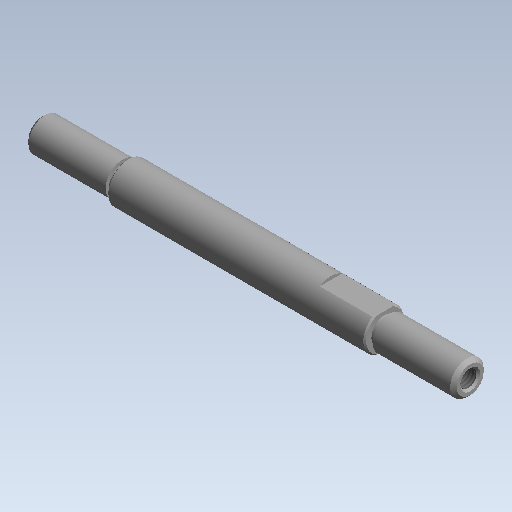
# Autodesk Inventor part: SSFRMHHS6-38.3-F12.7-P5-T12.7-M3-SC0-TF12.7-TT12.7
Saved by Autodesk Inventor 2020.3 (Build 243373000, 373)
## iProperties
Part Number: SSFRMHHS6-38.3-F12.7-P5-T12.7-M3-SC0-TF12.7-TT12.7
Material: 一般
Catalog Web Link: www.cadenas.de
Description: NSFRMHHS, SFRMHHS, PSFRMHHS, SSFRMHHS, NSFRMGHS, SFRMGHS, PSFRMGHS, SSFRMGHS, NSFRHHS, SFRHHS, PSFRHHS, SSFRHHS, NSFRHS, SFRHS, PSFRHS, SSFRHS_shaft-Rotary Shafts - Both Ends Stepped and Tapped - Wrench Flats
Vendor: MISUMI
Document SubType Name: Modeling
Designer: partserver
Manufacturer: MISUMI
Mass: 1.45427 g
Surface Area: 13.2412 cm^2
Volume: 1.45427 cm^3
Density: 1 g/cm^3
Appearance: PSOLRGB-192-192-192
Category: PARTsolutions
Company: MISUMI
PSOL_IDENT_0: {$CADENAS_DATA\23d-libs\misumi\metric\11_rotary_shafts\11_components\psfrhs\psfrhs.prj},734 {VTYP=3D
PSOL_IDENT_1: },{NB=SSFRMHHS6-38.3-F12.7-P5-T12.7-M3-SC0_s},{LINA=SSFRMHHS6-38.3-F12.7-P5-T12.7-M3-SC0},{NN=NSFRMH
PSOL_IDENT_2: HS, SFRMHHS, PSFRMHHS, SSFRMHHS, NSFRMGHS, SFRMGHS, PSFRMGHS, SSFRMGHS, NSFRHHS, SFRHHS, PSFRHHS, SS
PSOL_IDENT_3: FRHHS, NSFRHS, SFRHS, PSFRHS, SSFRHS_shaft},{DATE=11.03.2021 14:31:30},{GEOMDATE=16.02.2021 10:15:52
PSOL_IDENT_4: },{VERSION=},{LINEID=110},{WBVAR=TS,TYS,MAT,ST,ALT1,L,ALT9,F,T,P,M,SC,ALT2,KC,A,WKC,C,K,E,KZ,Z,ALT8,
PSOL_IDENT_5: PKC,ALT14,QKC,ALT21,PP,PK,ALT23,PV,PW,ALT22,QQ,QK,ALT24,QV,QW,ALT27,TL,TR,ALT28,TF,ALT29,TTALT29,ALT
PSOL_IDENT_6: 3,FC,GALT3,WFC,J,WALT3,V,ALT4,SFC,SG,AG,ALT25,PFC,LC,ALT26,QFC,RC,ALT5,UC,ALT31},{WBNUMERIC=L,F,T,P,
PSOL_IDENT_7: M,SC,KC,A,WKC,C,K,E,KZ,Z,PKC,QKC,PP,PK,PV,PW,QQ,QK,QV,QW,TL,TR,TF,TTALT29,FC,GALT3,WFC,J,WALT3,V,SFC
PSOL_IDENT_8: ,SG,AG,PFC,LC,QFC,RC,UC}  {NB=SSFRMHHS6-38.3-F12.7-P5-T12.7-M3-SC0_s},{LINA=SSFRMHHS6-38.3-F12.7-P5-
PSOL_IDENT_9: T12.7-M3-SC0},{KT=DUMMY},{PN=SSFRMHHS6-38.3-F12.7-P5-T12.7-M3-SC0},{TYPE=SSFRMHHS},{TS=M},{TSALG= 'M'
PSOL_IDENT_10: ,'h9 (Cold-drawn)','H','h7 (Ground)','','g6 (Ground)' },{TYS=H},{TYSALG= 'H' , 'h7' , '' , 'g6' },{T
PSOL_IDENT_11: YSS=H},{MAT=SUS304},{MATALG= 'S45C','S45C Equivalent', 'SUS304','SUS304' },{ST=-},{STALG= '-','-' },
PSOL_IDENT_12: {D=6},{ALT1=},{L=38.3},{LALG=[15:496/0.1]},{LMIN=15.000},{LMAX=496.000},{CIFL=2},{CIFL2=2},{ALT9=},{
PSOL_IDENT_13: ALT9ALG= '','N/A' },{ALT9PN=},{F=12.7},{FALG=[2:25/0.1]},{FMIN=2.000},{FMAX=25.000},{T=12.7},{TALG=[
PSOL_IDENT_14: 2:25/0.1]},{TMIN=2.000},{TMAX=25},{Y=63.700},{P=5},{PALG=[5]},{PMIN=5},{PMIN1=3},{PMIN2=5},{PMIN3=3}
PSOL_IDENT_15: ,{PMAX=5},{M=3.0},{MALG=2.6,3},{M26=2.6,},{M3=3},{M4=},{M5=},{M6=},{M8=},{M10=},{M12=},{M16=},{M20=}
PSOL_IDENT_16: ,{M24=},{M30=},{ML=11.5},{ML3D1=6},{ML3D2=11.5},{CIFM=0},{PITCH=0.5},{MPN=-M3},{CIFC=1},{CC=0.2},{SC=
PSOL_IDENT_17: 0},{SCALG=[0:30/1]},{SCMIN=0},{SCMAX=30},{W=5},{LL2=8},{CIFSC=2},{CUTSC=11},{YMAX=500},{CIFR=0},{CIF
PSOL_IDENT_18: R2=0},{ALT2=},{ALT2ALG= '', 'w/o Key Grooves','KC','with KC (Key Groove)','WKC','with WKC (Two Key G
PSOL_IDENT_19: rooves)','KCWKC','with KC + WKC (Three Key Grooves)','KZ','with KC + WKC + KZ (Four Key Grooves)' },
PSOL_IDENT_20: {ALT2PN=},{KC=0.0},{KCALG=[0]},{KCMIN=0.000},{KCMAX=0.000},{A=0.0},{AALG=[0]},{AMIN=2.000},{AMAX=0.0
PSOL_IDENT_21: 00},{WKC=0.0},{WKCALG=[0]},{WKCMIN=0.000},{WKCMAX=0.000},{C=0.0},{CALG=[0]},{CMIN=2.000},{CMAX=0.000
PSOL_IDENT_22: },{K=0.0},{KALG=[0]},{KMIN=0.000},{KMAX=34.300},{E=0.0},{EALG=[0]},{EMIN=2.000},{EMAX=36.300},{KZ=0.
PSOL_IDENT_23: 0},{KZALG=[0]},{KZMIN=40.300},{KZMAX=36.300},{Z=0.0},{ZALG=[0]},{ZMIN=2.000},{ZMAX=38.300},{BB=0},{B
PSOL_IDENT_24: BALT2=2.000},{TT=0.0},{TTALT2=1.200},{CIFKC=1.000},{CIFWKC=1.000},{CIFK=1.000},{CIFKZ=2.000},{PCUT=0
PSOL_IDENT_25: .000},{PCUT3D=0.000},{QCUT=0.000},{QCUT3D=0.000},{ALT8=},{ALT8ALG= '','Not applicable' },{ALT8PN=},{
PSOL_IDENT_26: PKC=0.0},{PKCALG=[0]},{PKCMIN=0.000},{PKCMAX=12.700},{BBALT8=0.0},{TTALT8=0.000},{ALT14=},{ALT14ALG=
PSOL_IDENT_27: '','Not applicable' },{ALT14PN=},{QKC=0.0},{QKCALG=[0]},{QKCMIN=0.000},{QKCMAX=12.700},{BBALT14=0.0
PSOL_IDENT_28: },{TTALT14=0.000},{ALT21=},{ALT21ALG= '','Not applicable' },{ALT21PN=},{PP=0.0},{PPALG=[0]},{PPMIN=0
PSOL_IDENT_29: .000},{PPMAX=12.700},{PK=0.0},{PKALG=[0]},{PKMIN=0.000},{PKMAX=12.700},{ALT23=},{ALT23ALG= '','Not a
PSOL_IDENT_30: pplicable' },{ALT23PN=},{PV=0.0},{PVALG=[0]},{PVMIN=2.000},{PVMAX=12.700},{PW=0.0},{PWALG=[0]},{PWMI
PSOL_IDENT_31: N=0.000},{PWMAX=12.700},{ALT22=},{ALT22ALG= '','Not applicable' },{ALT22PN=},{QQ=0.0},{QQALG=[0]},{Q
PSOL_IDENT_32: QMIN=0.000},{QQMAX=12.700},{QK=0.0},{QKALG=[0]},{QKMIN=0.000},{QKMAX=12.700},{ALT24=},{ALT24ALG= '','
PSOL_IDENT_33: Not applicable' },{ALT24PN=},{QV=0.0},{QVALG=[0]},{QVMIN=2.000},{QVMAX=12.700},{QW=0.0},{QWALG=[0]},
PSOL_IDENT_34: {QWMIN=0.000},{QWMAX=12.700},{TPKC=0.200},{TPKCPKC3D=0.000},{TPKCPP3D=0.000},{TPKCPV3D=0.000},{TQKC=
PSOL_IDENT_35: 0.200},{TQKCQKC3D=0.000},{TQKCQQ3D=0.000},{TQKCQV3D=0.000},{CIFPP=1.000},{CIFPV=2.000},{CIFQQ=1.000}
PSOL_IDENT_36: ,{CIFQV=2.000},{ALT27=},{ALT27ALG= '','w/o Retaining Ring Groove at D','TL','with TL (Retaining Ring
PSOL_IDENT_37: Groove at D)','TR','with TR (Retaining Ring Groove at D)','TLTR','with TL + TR (Retaining Ring Groo
PSOL_IDENT_38: ve at D)' },{ALT27PN=},{TL=0.0},{TLALG=[0]},{TLMIN=2},{TLMAX=0},{TR=0.0},{TRALG=[0]},{TRMIN=2},{TRMA
PSOL_IDENT_39: X=0},{DDALT27=0.0},{MMALT27=0.00},{MMALT27ALG=0.7},{ALT28=},{ALT28ALG= '','w/o TF (Retaining Ring Gr
PSOL_IDENT_40: oove at Step P)','TF','with TF (Retaining Ring Groove at Step P)' },{ALT28PN=},{TF=0.0},{TFALG=[0]},
PSOL_IDENT_41: {TFMIN=2.7},{TFMAX=10.7},{DDALT28=0.0},{MMALT28=0.00},{MMALT28ALG=0.7},{ALT29=},{ALT29ALG= '','w/o T
PSOL_IDENT_42: T (Retaining Ring Groove at Step Q)','TT','with TT (Retaining Ring Groove at Step Q)' },{ALT29PN=},{
PSOL_IDENT_43: TTALT29=0.0},{TTALT29ALG=[0]},{TTALT29MIN=2.7},{TTALT29MAX=10.7},{DDALT29=0.0},{MMALT29=0.00},{MMALT
PSOL_IDENT_44: 29ALG=0.7},{ALT3=},{ALT3ALG= '', 'w/o Set Screw Flat','FC','with FC (Adds a Set Screw Flat)','WFC','
PSOL_IDENT_45: with WFC (Adds Two Set Screw Flats)','FCWFC','with FC + WFC (Adds Three Set Screw Flats)' },{ALT3PN=
PSOL_IDENT_46: },{FC=0},{FCALG=[0]},{FCMIN=0.000},{FCMIN2=6.000},{FCMAX=37.000},{FCMAX2=23.300},{GALT3=0},{GALT3ALG=
PSOL_IDENT_47: [0]},{GALT3MIN=1},{GALT3MAX=38},{GALT3MAX2=32},{GALT3MAX3=35},{WFC=0},{WFCALG=[0]},{WFCMIN=0},{WFCMI
PSOL_IDENT_48: N2=2},{WFCMAX=34},{WFCMAX2=-3},{WFCMAX3=-4},{J=0},{JALG=[0]},{JMIN=1},{JMAX=35},{JMAX2=-2},{JMAX3=-6
PSOL_IDENT_49: },{WALT3=0},{WALT3ALG=[0]},{WALT3MIN=0},{WALT3MIN2=41},{WALT3MAX=35},{WALT3MAX2=35},{V=0},{VALG=[0]}
PSOL_IDENT_50: ,{VMIN=1},{VMAX=36},{VMAX2=36},{CIFFC=0},{CIFCUT=0},{ALT4=},{ALT4ALG= '', 'w/o SFC (2 Set Screw Flat
PSOL_IDENT_51: s (Angle Specified))', 'SFC'  , 'with SFC (2 Set Screw Flats (Angle Specified))'},{ALT4PN=},{SFC=0},
PSOL_IDENT_52: {SFCALG=[0]},{SFCMIN=0},{SFCMAX=37},{SG=0},{SGALG=[0]},{SGMIN=1},{SGMAX=38},{AG=0},{AGALG=[0]},{H=0}
PSOL_IDENT_53: ,{CIFSFC=0},{CUTSFC=0},{ALT25=},{ALT25ALG= '','w/o PFC (Set Screw Flat on Step P)','PFC','with PFC (
PSOL_IDENT_54: Set Screw Flat on Step P)' },{ALT25PN=},{PFC=0},{PFCALG=[0]},{PFCMN=0},{PFCMAX=11},{LC=0},{LCALG=[0]
PSOL_IDENT_55: },{LCMIN=1},{LCMAX=12},{HALT25=0.0},{ALT26=},{ALT26ALG= '','w/o QFC (Set Screw Flat on Step Q)','QFC'
PSOL_IDENT_56: ,'with QFC (Set Screw Flat on Step Q)' },{ALT26PN=},{QFC=0},{QFCALG=[0]},{QFCMIN=0},{QFCMAX=11},{RC=
PSOL_IDENT_57: 0},{RCALG=[0]},{RCMIN=1},{RCMAX=12},{HALT26=0.0},{ALT5=},{ALT5ALG= '', 'w/o UC (Slit Cam Groove)', '
PSOL_IDENT_58: UC', 'with UC (Slit Cam Groove)'},{ALT5PN=},{UC=0},{UCALG=[0]},{UCMIN=1},{UCMAX=33},{DD=0},{LL1=0},{
PSOL_IDENT_59: ALT31=},{ALT31ALG= '', 'w/o Tapped Depth','MD','with MD (Tapped Depth)' },{CIFALT31M=0.000},{ERRORPN=
PSOL_IDENT_60: },{ERRORMALT2=OK},{ERRORMALT3=OK},{ERRORMALT4=OK},{ERRORMALT5=OK},{ERRORMALT8=OK},{ERRORMALT14=OK},{
PSOL_IDENT_61: ERRORMALT21=OK},{ERRORMALT22=OK},{ERRORMALT23=OK},{ERRORMALT24=OK},{ERRORMALT25=OK},{ERRORMALT26=OK}
PSOL_IDENT_62: ,{ERRORMALT27=OK},{ERRORMALT28=OK},{ERRORMALT29=OK},{ERRORSCALT2=OK},{ERRORSCALT3=OK},{ERRORSCALT4=O
PSOL_IDENT_63: K},{ERRORSCALT5=OK},{ERRORSCALT27=OK},{ERRORALT23=OK},{ERRORALT24=OK},{ERRORALT25=OK},{ERRORALT28=OK
PSOL_IDENT_64: },{ERRORALT34=OK},{ERRORALT35=OK},{ERRORALT45=OK},{ERRORALT214=OK},{ERRORALT221=OK},{ERRORALT222=OK}
PSOL_IDENT_65: ,{ERRORALT223=OK},{ERRORALT224=OK},{ERRORALT225=OK},{ERRORALT226=OK},{ERRORALT227=OK},{ERRORALT228=O
PSOL_IDENT_66: K},{ERRORALT229=OK},{ERRORALT825=OK},{ERRORALT828=OK},{ERRORALT1426=OK},{ERRORALT1429=OK},{ERRORALT2
PSOL_IDENT_67: 125=OK},{ERRORALT2128=OK},{ERRORALT2226=OK},{ERRORALT2229=OK},{ERRORALT2325=OK},{ERRORALT2328=OK},{E
PSOL_IDENT_68: RRORALT2426=OK},{ERRORALT2429=OK},{ERRORALT2528=OK},{ERRORALT2629=OK},{ERRORALT327=OK},{ERRORALT427=
PSOL_IDENT_69: OK},{ERRORALT527=OK},{ALT2829=4}
NB: SSFRMHHS6-38.3-F12.7-P5-T12.7-M3-SC0_s
NN: NSFRMHHS, SFRMHHS, PSFRMHHS, SSFRMHHS, NSFRMGHS, SFRMGHS, PSFRMGHS, SSFRMGHS, NSFRHHS, SFRHHS, PSFRHHS, SSFRHHS, NSFRHS, SFRHS, PSFRHS, SSFRHS_shaft
NT: Rotary Shafts - Both Ends Stepped and Tapped - Wrench Flats
NBSYN: $PN._s
LINA: SSFRMHHS6-38.3-F12.7-P5-T12.7-M3-SC0
CATALOG: Misumi
PN: SSFRMHHS6-38.3-F12.7-P5-T12.7-M3-SC0
TS: h9 (Cold-drawn)
TYS: h7
MAT: SUS304
ST: -
D: 6
ALT1: w/o LKC (Changes L Tolerance)
L: 38.3
ALT9: N/A
F: 12.7
T: 12.7
P: 5
M: 3
SC: 0
W: 5
LL2: 8
YMAX: 500
ALT2: w/o Key Grooves
KC: 0
A: 0
WKC: 0
C: 0
K: 0
E: 0
KZ: 0
Z: 0
BB: 0
TT: 0
ALT8: Not applicable
PKC: 0
BBALT8: 0
TTALT8: 0
ALT14: Not applicable
QKC: 0
BBALT14: 0
TTALT14: 0
ALT21: Not applicable
PP: 0
PK: 0
ALT23: Not applicable
PV: 0
PW: 0
ALT22: Not applicable
QQ: 0
QK: 0
ALT24: Not applicable
QV: 0
QW: 0
ALT27: w/o Retaining Ring Groove at D
TL: 0
TR: 0
DDALT27: 0
MMALT27: 0
ALT28: w/o TF (Retaining Ring Groove at Step P)
TF: 0
DDALT28: 0
MMALT28: 0
ALT29: w/o TT (Retaining Ring Groove at Step Q)
TTALT29: 0
DDALT29: 0
MMALT29: 0
ALT3: w/o Set Screw Flat
FC: 0
GALT3: 0
WFC: 0
J: 0
WALT3: 0
V: 0
ALT4: w/o SFC (2 Set Screw Flats (Angle Specified))
SFC: 0
SG: 0
AG: 0
H: 0
ALT25: w/o PFC (Set Screw Flat on Step P)
PFC: 0
LC: 0
HALT25: 0
ALT26: w/o QFC (Set Screw Flat on Step Q)
QFC: 0
RC: 0
ALT5: w/o UC (Slit Cam Groove)
UC: 0
DD: 0
LL1: 0
ALT31: w/o Tapped Depth
SUPPLIER: MISUMI
ARTICLENO: SSFRMHHS6-38.3-F12.7-P5-T12.7-M3-SC0_s
BOMINFO: SSFRMHHS6-38.3-F12.7-P5-T12.7-M3-SC0
CREATOR: CADENAS GmbH
Title: SSFRMHHS6-38.3-F12.7-P5-T12.7-M3-SC0
Author: Cadenas PARTsolutions
Comments: Rotary Shafts - Both Ends Stepped and Tapped - Wrench Flats
Autodesk Inventor part; units mm, degrees
ref_plane "YZ Plane" through (0, 0, 0) normal (1, 0, 0) x (0, 1, 0)
ref_plane "XZ Plane" through (0, 0, 0) normal (0, 1, 0) x (-1, 0, 0)
ref_plane "XY Plane" through (0, 0, 0) normal (0, 0, 1) x (1, 0, 0)
sketch "Sketch_1" plane through (0, 0, 0) normal (0, 0, 1) x (1, 0, 0)
  line L0 (51, 0) -> (-12.7, 0)
  line L1 (-12.7, 0) -> (-12.7, 2)
  line L2 (-12.7, 2) -> (-12.2, 2.5)
  line L3 (-12.2, 2.5) -> (-0.2, 2.5)
  arc A0 (-0.2, 2.5) -> (0, 2.7) centre (-0.2, 2.7) ccw
  line L4 (0, 2.7) -> (0, 2.8)
  line L5 (0, 2.8) -> (0.2, 3)
  line L6 (0.2, 3) -> (38.1, 3)
  line L7 (38.1, 3) -> (38.3, 2.8)
  line L8 (38.3, 2.8) -> (38.3, 2.7)
  arc A1 (38.3, 2.7) -> (38.5, 2.5) centre (38.5, 2.7) ccw
  line L9 (38.5, 2.5) -> (50.5, 2.5)
  line L10 (50.5, 2.5) -> (51, 2)
  line L11 (51, 2) -> (51, 0)
  line L12 (51, 0) -> (-12.7, 0)
  line L13 (38.3, 2.7) -> (38.3, 2)
  line L14 (38.3, 2) -> (39, 2)
  line L15 (39, 2) -> (39, 2.5)
  line L16 (0, 2.7) -> (0, 2)
  line L17 (0, 2) -> (-0.7, 2)
  line L18 (-0.7, 2) -> (-0.7, 2.5)
  dimension "d17" = 0.7
  dimension "d18" = 2
  dimension "d20" = 0.7
  dimension "d21" = 2
  constraints: 38 end point, 6 vertical, 5 horizontal, 4 perpendicular, 4 point on circle, 2 centre point, 2 point on line, 24 other
  measures "d17" distance between parallel lines of L13 L15
  measures "d18" distance between parallel lines of L14 L0
  measures "d20" distance between parallel lines of L18 L16
  measures "d21" distance between parallel lines of L0 L17
revolve "Revolution1" add sketch "Sketch_1" angle 360 about axis through (51, 0, 0) along (1, 0, 0)
sketch "Sketch2" plane through (-12.7, 0, 0) normal (-1, 0, 0) x (0, 0, 1)
  point P0 (0, 0)
hole "Hole1" at (-12.7, 0, 0) direction (1, 0, 0) diameter 2.459 depth 10.7901 tip angle 120 countersink diameter 3 countersink angle 90 thread size "M3x0.5" class "6H" standard "ISO Metric profile"
sketch "Sketch3" plane through (51, 0, 0) normal (1, 0, 0) x (0, 0, -1)
  point P0 (0, 0)
hole "Hole2" at (51, 0, 0) direction (-1, 0, 0) diameter 2.459 depth 10.7901 tip angle 120 countersink diameter 3 countersink angle 90 thread size "M3x0.5" class "6H" standard "ISO Metric profile"
sketch "Sketch_28" plane through (0, 0, 0) normal (1, 0, 0) x (0, 0, -1)
  line L0 (-5, -6) -> (5, -6)
  line L1 (5, -6) -> (5, 3)
  line L2 (5, 3) -> (2.5, 3)
  line L3 (2.5, 3) -> (2.5, -3)
  line L4 (2.5, -3) -> (-2.5, -3)
  line L5 (-2.5, -3) -> (-2.5, 3)
  line L6 (-2.5, 3) -> (-5, 3)
  line L7 (-5, 3) -> (-5, -6)
  constraints: 16 end point
extrude "Extrusion1" cut sketch "Sketch_28" along normal mid plane 16
revolve "回転2" cut sketch "Sketch_1" angle 360 about axis through (51, 0, 0) along (-1, 0, 0) contours L15 L14 L13 A1 L9 | L3 A0 L16 L17 L18
body "Solid1"
